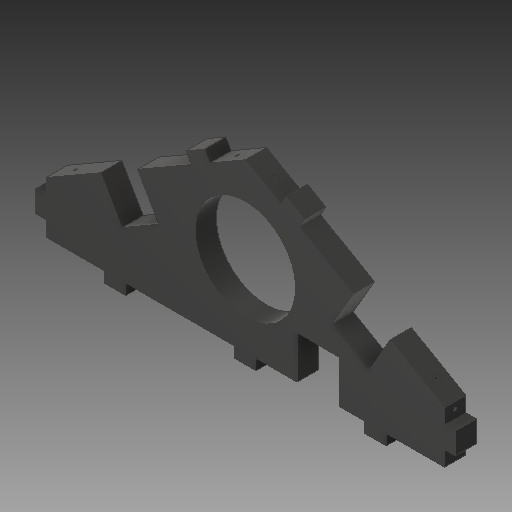
# Autodesk Inventor part: HB04
Saved by Autodesk Inventor 2017 (Build 210142000, 142)
## iProperties
Created: 2019-05-20
Part Number: HB04
Material: Polyethylene, High Density
Document SubType Name: Modeling
Designer: Dell
Density: 0.952 g/cm^3
Appearance: Smooth - Black
Mass: 1083.32 g
Surface Area: 1458.06 cm^2
Volume: 1137.95 cm^3
Author: Dell
Autodesk Inventor part; units mm, degrees
ref_plane "YZ Plane" through (0, 0, 0) normal (1, 0, 0) x (0, 1, 0)
ref_plane "XZ Plane" through (0, 0, 0) normal (0, 1, 0) x (-1, 0, 0)
ref_plane "XY Plane" through (0, 0, 0) normal (0, 0, 1) x (1, 0, 0)
sketch "Sketch1" plane through (0, 0, 0) normal (0, 0, 1) x (1, 0, 0)
  line L0 (262.89, 253.3796) -> (525.78, 101.6)
  line L1 (525.78, 101.6) -> (525.78, -201.9592) construction
  line L2 (525.78, -201.9592) -> (262.89, -353.7388) construction
  line L3 (262.89, -353.7388) -> (0, -201.9592) construction
  line L4 (0, -201.9592) -> (0, 101.6) construction
  line L5 (0, 101.6) -> (262.89, 253.3796)
  line L6 (0, 101.6) -> (0, 0)
  line L7 (0, 0) -> (525.78, 0)
  line L8 (525.78, 0) -> (525.78, 101.6)
  point P0 (262.89, -50.1796)
  dimension "d0" = 525.78
  dimension "d1" = 101.6
  constraints: 18 end point, 2 collinear, 2 point on line, 1 perpendicular, 1 vertical, 13 other
  measures "d0" distance between parallel lines of L4 L1
  measures "d1" distance of L6.end L4.end
extrude "Extrusion1" add sketch "Sketch1" along normal blind 25.4
sketch "Sketch2" plane through (0, 0, 25.4) normal (0, 0, 1) x (1, 0, 0)
  circle A0 centre (262.89, 121.3796) radius 60
  line L0 (0, 0) -> (525.78, 0) projected
  point P0 (262.89, 0)
  dimension "d4" = 121.3796
  dimension "d5" = 120
  constraints: 1 centre point, 1 midpoint, 1 vertical alignment
  measures "d4" distance from line of L0 A0.centre
  measures "d5" diameter of A0
extrude "Extrusion2" cut sketch "Sketch2" against normal through all
sketch "Sketch3" plane through (0, 0, 25.4) normal (0, 0, 1) x (1, 0, 0)
  circle A0 centre (262.89, 121.3796) radius 60 projected
  line L0 (0, 101.6) -> (0, 0) projected
  line L1 (0, 0) -> (525.78, 0) projected
  line L2 (525.78, 0) -> (525.78, 101.6) projected
  line L3 (525.78, 101.6) -> (262.89, 253.3796) projected
  line L4 (262.89, 253.3796) -> (0, 101.6) projected
  line L5 (25.4, 86.9353) -> (25.4, 25.4)
  line L6 (25.4, 25.4) -> (500.38, 25.4)
  line L7 (500.38, 25.4) -> (500.38, 86.9353)
  line L8 (500.38, 86.9353) -> (262.89, 224.0502)
  line L9 (262.89, 224.0502) -> (25.4, 86.9353)
  dimension "d8" = 25.4
  constraints: 10 end point, 4 other
  measures "d8" distance between parallel lines of L4 L9
extrude "Extrusion3" cut sketch "Sketch3" against normal through all contours L4 L3 L2 L1 L0
sketch "Sketch4" plane through (0, 0, 25.4) normal (0, 0, 1) x (1, 0, 0)
  line L0 (134.346, 149.8353) -> (159.746, 105.8412)
  line L1 (159.746, 105.8412) -> (115.7519, 80.4412)
  line L2 (115.7519, 80.4412) -> (90.3519, 124.4353)
  line L3 (90.3519, 124.4353) -> (134.346, 149.8353)
  line L4 (134.346, 149.8353) -> (115.7519, 80.4412) construction
  line L5 (159.746, 105.8412) -> (90.3519, 124.4353) construction
  line L6 (262.89, 224.0502) -> (25.4, 86.9353) projected
  line L7 (500.38, 86.9353) -> (262.89, 224.0502) projected
  line L8 (262.89, 224.0502) -> (262.89, 25.4)
  line L9 (25.4, 25.4) -> (500.38, 25.4) projected
  line L10 (391.434, 149.8353) -> (366.034, 105.8412)
  line L11 (366.034, 105.8412) -> (410.0281, 80.4412)
  line L12 (410.0281, 80.4412) -> (435.4281, 124.4353)
  line L13 (435.4281, 124.4353) -> (391.434, 149.8353)
  line L14 (391.434, 149.8353) -> (410.0281, 80.4412) construction
  line L15 (366.034, 105.8412) -> (435.4281, 124.4353) construction
  point P0 (0, 0)
  point P1 (125.049, 115.1383)
  point P2 (400.731, 115.1383)
  point P3 (381.635, 155.4928)
  dimension "d11" = 50.8
  dimension "d12" = 50.8
  dimension "d15" = 75
  constraints: 26 end point, 5 midpoint, 5 symmetric about line, 2 parallel, 1 perpendicular, 1 point on line
  measures "d11" distance of L2.end L0.start
  measures "d12" distance of L0.start L0.end
  measures "d15" distance from line of L6.end L2
extrude "Extrusion4" cut sketch "Sketch4" against normal through all
sketch "Sketch5" plane through (0, 0, 0) normal (0, 0, -1) x (-1, 0, 0)
  line L0 (-25.4, 86.9353) -> (-25.4, 25.4) projected
  line L1 (-25.4, 43.4677) -> (-12.7, 43.4677)
  line L2 (-12.7, 43.4677) -> (-12.7, 68.8677)
  line L3 (-12.7, 68.8677) -> (-25.4, 68.8677)
  line L4 (-25.4, 68.8677) -> (-25.4, 43.4677)
  line L5 (-25.4, 25.4) -> (-500.38, 25.4) projected
  line L6 (-94.99, 25.4) -> (-120.39, 25.4)
  line L7 (-120.39, 25.4) -> (-120.39, 12.7)
  line L8 (-120.39, 12.7) -> (-94.99, 12.7)
  line L9 (-94.99, 12.7) -> (-94.99, 25.4)
  line L10 (-405.39, 25.4) -> (-430.79, 25.4)
  line L11 (-430.79, 25.4) -> (-430.79, 12.7)
  line L12 (-430.79, 12.7) -> (-405.39, 12.7)
  line L13 (-405.39, 12.7) -> (-405.39, 25.4)
  line L14 (-500.38, 25.4) -> (-500.38, 86.9353) projected
  line L15 (-500.38, 43.4677) -> (-513.08, 43.4677)
  line L16 (-513.08, 43.4677) -> (-513.08, 68.8677)
  line L17 (-513.08, 68.8677) -> (-500.38, 68.8677)
  line L18 (-500.38, 68.8677) -> (-500.38, 43.4677)
  line L19 (-262.89, 224.0502) -> (-134.346, 149.8353) projected
  line L20 (-198.618, 186.9428) -> (-220.615, 199.6428)
  line L21 (-220.615, 199.6428) -> (-214.265, 210.6413)
  line L22 (-214.265, 210.6413) -> (-192.268, 197.9413)
  line L23 (-192.268, 197.9413) -> (-198.618, 186.9428)
  line L24 (-391.434, 149.8353) -> (-262.89, 224.0502) projected
  line L25 (-305.165, 199.6428) -> (-327.162, 186.9428)
  line L26 (-327.162, 186.9428) -> (-333.512, 197.9413)
  line L27 (-333.512, 197.9413) -> (-311.515, 210.6413)
  line L28 (-311.515, 210.6413) -> (-305.165, 199.6428)
  line L29 (-262.89, 224.0502) -> (-391.434, 149.8353) projected
  line L30 (-120.39, 19.05) -> (-405.39, 19.05) construction
  line L31 (-250.19, 25.4) -> (-275.59, 25.4)
  line L32 (-275.59, 25.4) -> (-275.59, 12.7)
  line L33 (-275.59, 12.7) -> (-250.19, 12.7)
  line L34 (-250.19, 12.7) -> (-250.19, 25.4)
  line L35 (-500.38, 25.4) -> (-25.4, 25.4) projected
  line L36 (-305.165, 199.6428) -> (-311.515, 210.6413)
  line L37 (-311.515, 210.6413) -> (-333.512, 197.9413)
  line L38 (-333.512, 197.9413) -> (-327.162, 186.9428)
  line L39 (-327.162, 186.9428) -> (-305.165, 199.6428)
  point P0 (0, 0)
  point P1 (-25.4, 56.1677)
  point P2 (-262.89, 25.4)
  point P3 (-262.89, 19.05)
  point P4 (-262.89, 25.4)
  dimension "d16" = 12.7
  dimension "d17" = 12.7
  dimension "d18" = 12.7
  dimension "d19" = 12.7
  dimension "d20" = 12.7
  dimension "d21" = 12.7
  dimension "d22" = 25.4
  dimension "d23" = 25.4
  dimension "d24" = 25.4
  dimension "d25" = 25.4
  dimension "d26" = 25.4
  dimension "d27" = 25.4
  dimension "d28" = 285
  dimension "d29" = 25.4
  dimension "d30" = 12.7
  constraints: 66 end point, 14 parallel, 10 midpoint, 8 point on line, 7 perpendicular, 5 horizontal, 4 collinear, 1 vertical alignment
  measures "d16" distance between parallel lines of L6 L8
  measures "d17" distance of L12.end L10.start
  measures "d18" distance of L15.start L15.end
  measures "d19" distance of L25.end L26.end
  measures "d20" distance of L20.end L21.end
  measures "d21" distance of L1.start L1.end
  measures "d22" distance of L7.end L8.end
  measures "d23" distance of L11.end L12.end
  measures "d24" distance of L1.end L2.end
  measures "d25" distance of L21.end L22.end
  measures "d26" distance of L26.end L27.end
  measures "d27" distance of L15.end L16.end
  measures "d28" distance of L30.start L30.end
  measures "d29" distance of L32.end L33.end
  measures "d30" distance of L31.end L32.end
extrude "Extrusion5" add sketch "Sketch5" against normal blind 25.4
sketch "Sketch6" plane through (0, 0, 0) normal (0, 0, -1) x (-1, 0, 0)
  line L0 (-275.59, 25.4) -> (-405.39, 25.4) projected
  line L1 (-324.58, 25.4) -> (-375.38, 25.4)
  line L2 (-375.38, 25.4) -> (-375.38, 76.2)
  line L3 (-375.38, 76.2) -> (-324.58, 76.2)
  line L4 (-324.58, 76.2) -> (-324.58, 25.4)
  line L5 (-500.38, 43.4677) -> (-500.38, 25.4) projected
  point P0 (0, 0)
  dimension "d33" = 50.8
  dimension "d34" = 50.8
  dimension "d35" = 125
  constraints: 8 end point, 2 parallel, 1 horizontal, 1 perpendicular, 1 point on line
  measures "d33" distance of L2.end L3.end
  measures "d34" distance of L1.end L2.end
  measures "d35" distance between parallel lines of L5 L2
extrude "Extrusion6" cut sketch "Sketch6" against normal through all
sketch "Sketch8" plane through (500.38, 86.9353, 25.4) normal (0.5, 0.866, 0) x (0.866, -0.5, 0)
  circle A0 centre (-248.8298, 12.7) radius 2
  circle A1 centre (-25.4, 12.7) radius 2
  line L0 (0, 0) -> (0, 25.4) projected
  line L1 (-274.2298, 0) -> (-274.2298, 25.4) projected
  point P0 (-389.8741, 25.4)
  point P1 (0, 12.7)
  dimension "d44" = 4
  dimension "d45" = 4
  dimension "d46" = 25.4
  dimension "d47" = 25.4
  constraints: 2 centre point, 2 horizontal alignment, 1 midpoint
  measures "d44" diameter of A0
  measures "d45" diameter of A1
  measures "d46" distance from line of L0 A1.centre
  measures "d47" distance from line of L1 A0.centre
extrude "Extrusion8" cut sketch "Sketch8" against normal blind 38.1
sketch "Sketch9" plane through (262.89, 224.0502, 25.4) normal (-0.5, 0.866, 0) x (0.866, 0.5, 0)
  line L0 (0, 0) -> (0, 25.4) projected
  line L1 (-274.2298, 0) -> (-274.2298, 25.4) projected
  circle A0 centre (-25.4, 12.7) radius 2
  circle A1 centre (-248.8298, 12.7) radius 2
  point P0 (-339.6945, 25.4)
  point P1 (-274.2298, 12.7)
  dimension "d50" = 4
  dimension "d51" = 4
  dimension "d52" = 25.4
  dimension "d53" = 25.4
  constraints: 2 centre point, 2 horizontal alignment, 1 midpoint
  measures "d50" diameter of A0
  measures "d51" diameter of A1
  measures "d52" distance from line of L1 A1.centre
  measures "d53" distance from line of L0 A0.centre
extrude "Extrusion9" cut sketch "Sketch9" against normal blind 38.1
sketch "Sketch10" plane through (500.38, 25.4, 25.4) normal (1, 0, 0) x (0, 0, -1)
  line L0 (0, 0) -> (25.4, 0) projected
  line L1 (0, 61.5353) -> (25.4, 61.5353) projected
  circle A0 centre (12.7, 8) radius 2
  circle A1 centre (12.7, 53.5353) radius 2
  point P0 (25.4, -25.4)
  point P1 (12.7, 0)
  point P2 (12.7, 61.5353)
  dimension "d56" = 4
  dimension "d57" = 4
  dimension "d58" = 8
  dimension "d59" = 8
  constraints: 2 centre point, 2 midpoint, 2 vertical alignment
  measures "d56" diameter of A0
  measures "d57" diameter of A1
  measures "d58" distance from line of L0 A0.centre
  measures "d59" distance from line of L1 A1.centre
extrude "Extrusion10" cut sketch "Sketch10" against normal blind 38.1
sketch "Sketch11" plane through (25.4, 86.9353, 0) normal (-1, 0, 0) x (0, 0, 1)
  circle A0 centre (12.7, -8) radius 2 projected
  circle A1 centre (12.7, -53.5353) radius 2 projected
  point P0 (0, -86.9353)
extrude "Extrusion11" cut sketch "Sketch11" against normal blind 38.1
sketch "Sketch12" plane through (120.39, 25.4, 25.4) normal (0, -1, 0) x (1, 0, 0)
  circle A0 centre (-60.195, -12.7) radius 2
  circle A1 centre (64.9, -12.7) radius 2
  circle A2 centre (345.195, -12.7) radius 2
  line L0 (310.4, 0) -> (379.99, 0) projected
  line L1 (0, 0) -> (129.8, 0) projected
  line L2 (-94.99, 0) -> (-25.4, 0) projected
  line L3 (379.99, 0) -> (379.99, -25.4) projected
  point P0 (-120.39, -25.4)
  point P1 (345.195, 0)
  point P2 (64.9, 0)
  point P3 (-60.195, 0)
  point P4 (379.99, -12.7)
  dimension "d64" = 4
  dimension "d65" = 4
  dimension "d66" = 4
  constraints: 4 midpoint, 3 centre point, 3 horizontal alignment, 3 vertical alignment
  measures "d64" diameter of A0
  measures "d65" diameter of A1
  measures "d66" diameter of A2
extrude "Extrusion12" cut sketch "Sketch12" against normal blind 38.1
body "Solid1"
